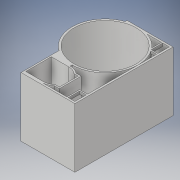
# Autodesk Inventor part: BoitCase
Saved by Autodesk Inventor 2019 (Build 230136000, 136)
## iProperties
Created: 2019-04-08
Part Number: BoitCase
Material: Generic
Document SubType Name: Modeling
Designer: Jorian Brusind
Density: 1 g/cm^3
Appearance: Default
Author: Jorian Brusind
Autodesk Inventor part; units mm, degrees
ref_plane "YZ Plane" through (0, 0, 0) normal (1, 0, 0) x (0, 1, 0)
ref_plane "XZ Plane" through (0, 0, 0) normal (0, 1, 0) x (-1, 0, 0)
ref_plane "XY Plane" through (0, 0, 0) normal (0, 0, 1) x (1, 0, 0)
sketch "Sketch7" plane through (0, 0, 0) normal (0, 1, 0) x (-1, 0, 0)
  line L0 (0, 0) -> (74, 0)
  line L1 (74, 0) -> (74, -104)
  line L2 (74, -104) -> (0, -104)
  line L3 (0, -104) -> (0, 0)
  dimension "d50" = 74
  dimension "d51" = 104
  constraints: 8 end point, 2 parallel, 1 horizontal, 1 perpendicular
  measures "d50" distance of L1.end L2.end
  measures "d51" distance of L0.end L1.end
extrude "Extrusion6" add sketch "Sketch7" along normal blind 3
sketch "Sketch8" plane through (0, 3, 0) normal (0, 1, 0) x (1, 0, 0)
  line L0 (0, 0) -> (0, 2)
  line L1 (0, 0) -> (0, 104) projected
  line L2 (0, 2) -> (-2, 2)
  line L3 (-2, 2) -> (-72, 2)
  line L4 (-72, 2) -> (-72, 102)
  line L5 (-72, 102) -> (-2, 102)
  line L6 (-2, 102) -> (-2, 2)
  line L7 (0, 104) -> (-74, 104) projected
  line L8 (0, 0) -> (-74, 0)
  line L9 (-74, 0) -> (-74, 104)
  line L10 (-74, 104) -> (0, 104)
  line L11 (0, 104) -> (0, 0)
  dimension "d54" = 2
  dimension "d55" = 2
  dimension "d56" = 70
  dimension "d57" = 100
  constraints: 20 end point, 4 parallel, 3 perpendicular, 2 horizontal, 1 point on line
  measures "d54" distance of L0.start L0.end
  measures "d55" distance of L0.end L2.end
  measures "d56" distance of L4.end L5.end
  measures "d57" distance of L3.end L4.end
extrude "Extrusion7" add sketch "Sketch8" along normal blind 60
sketch "Sketch9" plane through (0, 63, 0) normal (0, 1, 0) x (1, 0, 0)
  line L0 (-2, 102) -> (-72, 102) projected
  line L1 (-2, 102) -> (-37, 102)
  line L2 (-37, 102) -> (-37, 69)
  circle A0 centre (-37, 69) radius 33
  circle A1 centre (-37, 69) radius 35
  line L3 (-72, 102) -> (-72, 2) projected
  point P0 (0, 0)
  dimension "d60" = 35
  dimension "d61" = 33
  dimension "d62" = 66
  constraints: 4 end point, 2 centre point, 2 coincident, 1 midpoint, 1 perpendicular, 1 tangent
  measures "d60" distance of L0.start L1.end
  measures "d61" distance of L1.end L2.end
  measures "d62" diameter of A0
extrude "Extrusion8" add sketch "Sketch9" against normal blind 60 contours A1 L0 | L0 A1
sketch "Sketch10" plane through (0, 63, 0) normal (0, 1, 0) x (1, 0, 0)
  line L0 (-2, 2) -> (-72, 2) projected
  line L1 (-2, 2) -> (-37, 2)
  line L2 (-37, 2) -> (-37, 17)
  line L3 (-23.5, 17) -> (-23.5, 27)
  line L4 (-23.5, 17) -> (-23.5, 7)
  line L5 (-23.5, 7) -> (-27.9308, 7)
  line L6 (-23.5, 27) -> (-27.9308, 27)
  line L7 (-37, 3.5) -> (-55.5, 3.5)
  line L8 (-37, 30.5) -> (-55.5, 30.5)
  line L9 (-55.5, 30.5) -> (-55.5, 3.5)
  arc A0 (-37, 3.5) -> (-27.9308, 7) centre (-37, 17) ccw
  arc A1 (-27.9308, 27) -> (-37, 30.5) centre (-37, 17) ccw
  line L10 (-57.1, 1.9) -> (-37, 1.9)
  arc A2 (-37, 1.9) -> (-27.333, 5.4) centre (-37, 17) ccw
  line L11 (-27.333, 5.4) -> (-21.9, 5.4)
  line L12 (-21.9, 5.4) -> (-21.9, 17)
  line L13 (-21.9, 17) -> (-21.9, 28.6)
  line L14 (-21.9, 28.6) -> (-27.333, 28.6)
  arc A3 (-27.333, 28.6) -> (-37, 32.1) centre (-37, 17) ccw
  line L15 (-37, 32.1) -> (-57.1, 32.1)
  line L16 (-57.1, 32.1) -> (-57.1, 1.9)
  point P0 (0, 0)
  dimension "d65" = 35
  dimension "d66" = 15
  dimension "d68" = 10
  dimension "d69" = 10
  dimension "d70" = 18.5
  dimension "d71" = 13.5
  dimension "d72" = 13.5
  dimension "d73" = 4.4308
  dimension "d74" = 1.6
  constraints: 32 end point, 8 point on circle, 4 centre point, 4 tangent, 3 perpendicular, 3 vertical, 2 horizontal, 2 parallel, 1 coincident, 1 midpoint, 1 point on line, 8 other
  measures "d65" distance of L0.start L1.end
  measures "d66" distance of L1.end L2.end
  measures "d68" distance of L3.start L3.end
  measures "d69" distance of L3.start L4.end
  measures "d70" distance of L7.start L7.end
  measures "d71" radius of A1
  measures "d72" radius of A0
  measures "d73" distance of L4.end L5.end
  measures "d74" distance between parallel lines of L9 L16
extrude "Extrusion9" add sketch "Sketch10" against normal blind 60
sketch "Sketch11" plane through (0, 63, 0) normal (0, 1, 0) x (1, 0, 0)
  line L0 (-72, 2) -> (-57.1, 2) projected
  line L1 (-57.1, 2) -> (-57.1, 0)
  line L2 (-57.1, 2) -> (-57.1, 40.3471)
  arc A0 (-72, 69) -> (-2, 69) centre (-37, 69) ccw projected
  line L3 (-74, 0) -> (0, 0) projected
  line L4 (-57.1, 0) -> (-74, 0)
  line L5 (-74, 0) -> (-74, 104) projected
  arc A1 (-48.6619, 102) -> (-72, 69) centre (-37, 69) ccw projected
  line L6 (-74, 0) -> (-74, 69)
  arc A2 (-72, 69) -> (-57.1, 40.3471) centre (-37, 69) ccw
  arc A3 (-2, 69) -> (-25.3381, 102) centre (-37, 69) ccw projected
  line L7 (0, 0) -> (0, 104) projected
  circle A4 centre (-37, 69) radius 33 projected
  line L8 (-74, 104) -> (-74, 0) projected
  line L9 (-74, 69) -> (-74, 104)
  line L10 (-48.6619, 102) -> (-48.6619, 104)
  line L11 (0, 104) -> (-74, 104) projected
  line L12 (-48.6619, 104) -> (-74, 104)
  arc A5 (-48.6619, 102) -> (-72, 69) centre (-37, 69) ccw
  constraints: 14 end point, 5 point on circle, 4 collinear, 3 vertical, 2 centre point, 2 coincident, 1 point on line
extrude "Extrusion11" cut sketch "Sketch11" against normal blind 63 contours L1 L3 L5 L11 L10 A1 A0 L2
sketch "Sketch12" plane through (0, 63, 0) normal (0, 1, 0) x (1, 0, 0)
  line L0 (-2, 2) -> (-2, 69) projected
  line L1 (-2, 102) -> (-2, 69) projected
  line L2 (-2, 102) -> (-9, 102)
  line L3 (-9, 102) -> (-9, 90)
  line L4 (-9, 90) -> (-2, 90)
  line L5 (-2, 90) -> (-2, 102)
  line L6 (-9, 90) -> (-10.4295, 88.5705)
  circle A0 centre (-37, 69) radius 33 projected
  line L7 (-9, 90) -> (-6.9784, 90) construction
  line L8 (-10.4295, 88.5705) -> (-0.5715, 88.5705)
  line L9 (-0.5715, 88.5705) -> (-0.5715, 103.4285)
  line L10 (-0.5715, 103.4285) -> (-10.4295, 103.4285)
  line L11 (-10.4295, 103.4285) -> (-10.4295, 88.5705)
  line L12 (-2, 2) -> (-9, 2)
  line L13 (-9, 2) -> (-9, 14)
  line L14 (-9, 14) -> (-2, 14)
  line L15 (-2, 14) -> (-2, 2)
  line L16 (-10.429, 15.429) -> (-10.429, 0.571)
  line L17 (-10.429, 0.571) -> (-0.571, 0.571)
  line L18 (-0.571, 0.571) -> (-0.571, 15.429)
  line L19 (-0.571, 15.429) -> (-10.429, 15.429)
  point P0 (0, 0)
  dimension "d86" = 7
  dimension "d87" = 12
  dimension "d88" = 135
  dimension "d89" = 9.858
  dimension "d90" = 14.858
  dimension "d91" = 7
  dimension "d92" = 12
  dimension "d93" = 1.429
  constraints: 36 end point, 8 parallel, 4 horizontal, 4 perpendicular, 1 equal length, 5 other
  measures "d86" distance of L4.end L3.end
  measures "d87" distance of L3.end L2.end
  measures "d88" angle of L6 L7
  measures "d89" distance of L10.end L9.end
  measures "d90" distance of L9.end L8.end
  measures "d91" distance of L13.end L14.end
  measures "d92" distance of L12.end L13.end
  measures "d93" distance between parallel lines of L13 L16
extrude "Extrusion12" add sketch "Sketch12" against normal blind 3 contours L2 L3 L6 L11 L10 L9 L8 L1 | L1 L8 L6 L4 | L19 L18 L17 L16
pattern_linear "Rectangular Pattern1" count 3 spacing 20 along (0, -1, 0) of "Extrusion12"
sketch "Sketch13" plane through (0, 63, 0) normal (0, 1, 0) x (1, 0, 0)
  line L0 (-57.1, 32.1) -> (-37, 32.1) projected
  line L1 (-57.1, 0) -> (-57.1, 40.3471) projected
  line L2 (-57.1, 32.1) -> (-57.1, 40.3471)
  line L3 (-57.1, 32.1) -> (-37, 32.1)
  line L4 (-37, 32.1) -> (-37, 34)
  arc A0 (-57.1, 40.3471) -> (-2, 69) centre (-37, 69) ccw projected
  arc A1 (-57.1, 40.3471) -> (-37, 34) centre (-37, 69) ccw
  point P0 (0, 0)
  constraints: 6 end point, 3 point on circle, 2 collinear, 1 centre point, 1 coincident, 1 perpendicular
extrude "Extrusion13" add sketch "Sketch13" against normal blind 60
sketch "Sketch14" plane through (-55.5, 63, -30.5) normal (0, 0, 1) x (1, 0, 0)
  line L0 (-1.6, -63) -> (-1.6, -60)
  line L1 (-1.6, 0) -> (-1.6, -63) projected
  line L2 (-1.6, -60) -> (3.65, -60)
  line L3 (0, -60) -> (18.5, -60) projected
  line L4 (3.65, -60) -> (11.65, -60)
  line L5 (11.65, -60) -> (11.65, -56)
  line L6 (11.65, -56) -> (3.65, -56)
  line L7 (3.65, -56) -> (3.65, -60)
  point P0 (55.5, -63)
  dimension "d101" = 3
  dimension "d102" = 5.25
  dimension "d103" = 8
  dimension "d104" = 4
  constraints: 12 end point, 2 parallel, 2 point on line, 1 horizontal, 1 perpendicular
  measures "d101" distance of L0.start L0.end
  measures "d102" distance of L0.end L2.end
  measures "d103" distance of L6.end L5.end
  measures "d104" distance of L5.end L4.end
extrude "Extrusion14" cut sketch "Sketch14" against normal blind 9
body "Solid2"
